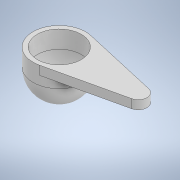
# Autodesk Inventor part: powderScoop
Saved by Autodesk Inventor 2022.3 (Build 263350030, 350C)
## iProperties
Created: 2022-09-24
Part Number: powderScoop
Material: Generic
Document SubType Name: Modeling
Designer: yiunf
Density: 1 g/cm^3
Appearance: Default
Author: yiunf
## iProperties of the stored document powderScoop_3DPrint.ipt
Created: 2022-09-24
Part Number: powderScoop_3DPrint
Material: Generic
Document SubType Name: Modeling
Designer: yiunf
Density: 1 g/cm^3
Appearance: Default
Author: yiunf
Autodesk Inventor part; units mm, degrees
ref_plane "YZ Plane" through (0, 0, 0) normal (1, 0, 0) x (0, 1, 0)
ref_plane "XZ Plane" through (0, 0, 0) normal (0, 1, 0) x (-1, 0, 0)
ref_plane "XY Plane" through (0, 0, 0) normal (0, 0, 1) x (1, 0, 0)
sketch "Sketch2" plane through (0, 0, 0) normal (0, 1, 0) x (-1, 0, 0)
  circle A0 centre (0, 0) radius 6.269
  circle A1 centre (0, 0) radius 7.5
  dimension "d0" = 12.538
  dimension "d1" = 15
  constraints: 2 centre point, 2 coincident
  measures "d0" diameter of A0
  measures "d1" diameter of A1
extrude "Extrusion1" add sketch "Sketch2" along normal blind 5
sketch "Sketch4" plane through (0, 5, 0) normal (0, 1, 0) x (1, 0, 0)
  circle A0 centre (0, 0) radius 7.5 projected
  circle A1 centre (0, 0) radius 6.269 projected
  circle A2 centre (0, 0) radius 7.5 projected
  line L0 (7.5, 0) -> (22.5, 0)
  circle A3 centre (22.5, 0) radius 2.5
  line L1 (22.97, -2.457) -> (1.6667, -7.3125)
  line L2 (22.97, 2.457) -> (1.6667, 7.3125)
  line L3 (22.97, -2.457) -> (23.0556, -2.4375)
  line L4 (22.97, 2.457) -> (23.0556, 2.4375)
  point P0 (22.5114, 2.4471)
  point P1 (1.6667, 7.3125)
  point P2 (1.6667, -7.3125)
  point P3 (22.5114, -2.4471)
  dimension "d11" = 15
  dimension "d12" = 5
  constraints: 10 end point, 4 point on circle, 3 tangent, 2 symmetric about line, 1 centre point, 1 coincident, 1 horizontal, 1 point on line
  measures "d11" distance of L0.start L0.end
  measures "d12" diameter of A3
extrude "Extrusion3" add sketch "Sketch4" against normal blind 2.5 contours L0 A3 L1 A0 | A0 L2 A3 L0 | A3
sketch "Sketch5" plane through (0, 0, 0) normal (0, -1, 0) x (1, 0, 0)
  circle A0 centre (0, 0) radius 7.5 projected
  circle A1 centre (0, 0) radius 6.269 projected
  line L0 (0, 7.5) -> (0, -7.5)
  circle A2 centre (0, 0) radius 7.5 projected
  point P0 (0, -6.269)
  point P1 (0, -7.5)
  point P2 (0, 6.269)
  constraints: 2 end point, 1 point on circle, 1 vertical, 2 other
revolve "Revolution2" add sketch "Sketch5" angle 180 about axis through (0, 0, 7.5) along (0, 0, -1) picked at (6.9746, -1.0213) contours A0 L0 A1
body "Solid1"
